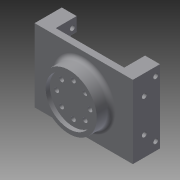
# Autodesk Inventor part: 90turnmount
Saved by Autodesk Inventor 2015 (Build 190159000, 159)
## iProperties
Created: 2016-12-16
Part Number: 90turnmount
Material: Generic
Document SubType Name: Modeling
Designer: Rudge-Top
Density: 1 g/cm^3
Appearance: Default
Author: Rudge-Top
Autodesk Inventor part; units mm, degrees
ref_plane "YZ Plane" through (0, 0, 0) normal (1, 0, 0) x (0, 1, 0)
ref_plane "XZ Plane" through (0, 0, 0) normal (0, 1, 0) x (-1, 0, 0)
ref_plane "XY Plane" through (0, 0, 0) normal (0, 0, 1) x (1, 0, 0)
sketch "Sketch1" plane through (0, 0, 0) normal (0, 1, 0) x (-1, 0, 0)
  circle A0 centre (0, 0) radius 11.25
  circle A1 centre (0, 0) radius 13.25
  dimension "d0" = 22.5
  dimension "d1" = 26.5
  constraints: 2 centre point, 2 coincident
  measures "d0" diameter of A0
  measures "d1" diameter of A1
extrude "Extrusion1" add sketch "Sketch1" along normal blind 2
sketch "Sketch2" plane through (0, 2, 0) normal (0, 1, 0) x (1, 0, 0)
  circle A0 centre (0, 0) radius 11.25 projected
  circle A1 centre (0, 0) radius 13.25 projected
extrude "Extrusion2" add sketch "Sketch2" along normal blind 5 contours A0 | A1
sketch "Sketch3" plane through (0, 7, 0) normal (0, 1, 0) x (1, 0, 0)
  line L0 (23.55, -17.5) -> (-23.55, -17.5)
  line L1 (-23.55, -17.5) -> (-23.55, 17.5)
  line L2 (-23.55, 17.5) -> (23.55, 17.5)
  line L3 (23.55, 17.5) -> (23.55, -17.5)
  point P0 (0, 0)
  dimension "d6" = 47.1
  dimension "d7" = 35
  dimension "d8" = 17.5
  dimension "d9" = 23.55
  constraints: 8 end point, 2 parallel, 1 horizontal, 1 perpendicular
  measures "d6" distance of L1.end L2.end
  measures "d7" distance of L2.end L0.start
  measures "d8" distance from line of L0 point (0, 0)
  measures "d9" distance from line of point (0, 0) L3
extrude "Extrusion3" add sketch "Sketch3" along normal blind 3
fillet "Fillet1" radius 2 1 edges at (-13.25, 7, 0)
sketch "Sketch4" plane through (0, 10, 0) normal (0, 1, 0) x (1, 0, 0)
  line L0 (-23.55, 17.5) -> (23.55, 17.5) projected
  line L1 (23.55, -17.5) -> (16.4, -17.5)
  line L2 (16.4, -17.5) -> (16.4, 17.5)
  line L3 (16.4, 17.5) -> (23.55, 17.5)
  line L4 (23.55, 17.5) -> (23.55, -17.5)
  line L5 (-23.55, -17.5) -> (-16.4, -17.5)
  line L6 (-16.4, -17.5) -> (-16.4, 17.5)
  line L7 (-16.4, 17.5) -> (-23.55, 17.5)
  line L8 (-23.55, 17.5) -> (-23.55, -17.5)
  point P0 (0, 0)
  dimension "d13" = 7.15
  dimension "d14" = 7.15
  constraints: 16 end point, 4 parallel, 2 horizontal, 2 perpendicular, 2 point on line
  measures "d13" distance of L2.end L3.end
  measures "d14" distance of L7.end L6.end
extrude "Extrusion4" add sketch "Sketch4" along normal blind 10
sketch "Sketch5" plane through (23.55, 7, 17.5) normal (1, 0, 0) x (0, 0, -1)
  line L0 (35, 0) -> (0, 0) projected
  line L1 (35, 0) -> (35, 13) projected
  line L2 (0, 13) -> (35, 13) projected
  line L3 (0, 0) -> (0, 13) projected
  line L4 (35, 13) -> (0, 13) projected
  line L5 (17.5, 13) -> (17.5, 7.9729)
  point P0 (17.5, -7)
  point P1 (25.5, 5.5)
  point P2 (31, 11)
  point P3 (9.5, 5.5)
  point P4 (4, 11)
  dimension "d17" = 5.5
  dimension "d18" = 5.5
  dimension "d19" = 8
  dimension "d20" = 13.5
  constraints: 2 end point, 2 symmetric about line, 1 midpoint, 1 vertical
  measures "d17" distance from line of L0 point (25.5, 5.5)
  measures "d18" horizontal distance of point (31, 11) point (25.5, 5.5)
  measures "d19" distance from line of L5 point (25.5, 5.5)
  measures "d20" distance from line of L5 point (31, 11)
hole "Hole1" at (23.55, 12.5, -8) at (23.55, 18, -13.5) at (23.55, 18, 13.5) at (23.55, 12.5, 8) direction (-1, 0, 0) diameter 2.3 end through all
sketch "Sketch6" plane through (0, 20, 0) normal (0, 1, 0) x (1, 0, 0)
  line L0 (23.55, -17.5) -> (23.55, 17.5) projected
  line L1 (23.55, 17.5) -> (16.4, 17.5) projected
  line L2 (16.4, 17.5) -> (16.4, -17.5) projected
  line L3 (16.4, -17.5) -> (23.55, -17.5) projected
  line L4 (16.4, 17.5) -> (16.4, -17.5) projected
  line L5 (16.4, -10.5) -> (19.3, -10.5)
  line L6 (19.3, -10.5) -> (19.3, 10.5)
  line L7 (19.3, 10.5) -> (16.4, 10.5)
  line L8 (16.4, 10.5) -> (16.4, -10.5)
  point P0 (0, 0)
  dimension "d28" = 2.9
  dimension "d29" = 21
  dimension "d30" = 7
  constraints: 8 end point, 2 parallel, 1 horizontal, 1 perpendicular, 1 point on line
  measures "d28" distance of L7.end L6.end
  measures "d29" distance of L6.end L5.end
  measures "d30" distance between parallel lines of L5 L3
extrude "Extrusion5" cut sketch "Sketch6" against normal blind 5.1 contours L2 L7 L6 L5
sketch "Sketch7" plane through (0, 20, 0) normal (0, 1, 0) x (1, 0, 0)
  line L0 (-16.4, 17.5) -> (-23.55, 17.5) projected
  line L1 (-23.55, 17.5) -> (-23.55, -17.5) projected
  line L2 (-23.55, -17.5) -> (-16.4, -17.5) projected
  line L3 (-16.4, -17.5) -> (-16.4, 17.5) projected
  line L4 (-16.4, -10.6) -> (-19.3, -10.6)
  line L5 (-19.3, -10.6) -> (-19.3, -3.6)
  line L6 (-19.3, -3.6) -> (-16.4, -3.6)
  line L7 (-16.4, -3.6) -> (-16.4, -10.6)
  line L8 (-16.4, 10.6) -> (-19.3, 10.6)
  line L9 (-19.3, 10.6) -> (-19.3, 3.6)
  line L10 (-19.3, 3.6) -> (-16.4, 3.6)
  line L11 (-16.4, 3.6) -> (-16.4, 10.6)
  point P0 (0, 0)
  dimension "d33" = 2.9
  dimension "d34" = 7
  dimension "d35" = 6.9
  dimension "d36" = 2.9
  dimension "d37" = 7
  dimension "d38" = 6.9
  constraints: 16 end point, 4 parallel, 2 horizontal, 2 perpendicular, 2 point on line
  measures "d33" distance of L5.end L6.end
  measures "d34" distance of L4.end L5.end
  measures "d35" distance between parallel lines of L2 L4
  measures "d36" distance of L10.end L9.end
  measures "d37" distance of L9.end L8.end
  measures "d38" distance between parallel lines of L0 L8
extrude "Extrusion6" cut sketch "Sketch7" against normal blind 5.1 contours L3 L10 L9 L8 | L3 L4 L5 L6
fillet "Fillet2" radius 0.5 9 edges at (-16.4, 17.45, 10.6) (-16.4, 14.9, 7.1) (-16.4, 17.45, 3.6) (-16.4, 14.9, -7.1) (-16.4, 17.45, -3.6) (-16.4, 17.45, -10.6) (16.4, 17.45, 10.5) (16.4, 14.9, 0) (16.4, 17.45, -10.5)
sketch "Sketch8" plane through (0, 2, 0) normal (0, -1, 0) x (1, 0, 0)
  point P0 (0, 0)
  point P1 (0, -8)
  point P2 (5.6569, -5.6569)
  point P3 (8, 0)
  point P4 (5.6569, 5.6569)
  point P5 (0, 8)
  point P6 (-5.6569, 5.6569)
  point P7 (-8, 0)
  point P8 (-5.6569, -5.6569)
  dimension "d42" = 8
  dimension "d45" = 360
  constraints: 9 other
  measures "d42" distance of point (0, 0) point (0, -8)
hole "Hole2" at (0, 2, -8) at (5.6569, 2, -5.6569) at (8, 2, 0) at (5.6569, 2, 5.6569) at (0, 2, 8) at (-5.6569, 2, 5.6569) at (-8, 2, 0) at (-5.6569, 2, -5.6569) direction (0, 1, 0) diameter 2.3 end through all
body "Solid1"
